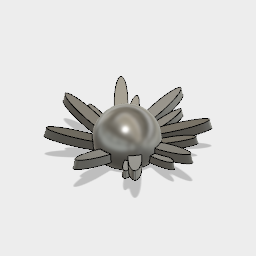
FPROJ_5 (Autodesk Fusion 360 design; units mm, degrees)
Autodesk Fusion 360 part; units mm, degrees
sketch "草图1" plane through (0, 0, 0) normal (0, 1, 0) x (1, 0, 0)
  ellipse E0 centre (0, 0) end of major axis (10, 0) minor radius 2
  line L0 (-10, 0) -> (10, 0)
  line L1 (0, -2) -> (0, 2)
extrude "拉伸1" add sketch "草图1" along normal blind 3 makes body 1
move_body "移动1" bodies 1 to x (0.965926, 0.258819, 0) y (-0.258819, 0.965926, 0) z (0, 0, 1) at (-0.3407, 2.5882, 0)
box "长方体基本要素1" add length 6 width 6 height 6 placed x (0, 1, 0) y (0, 0, 1) z (1, 0, 0) at (0, -45, -4) separate body makes body 2
move_body "移动2" bodies 2 to x (1, 0, 0) y (0, 1, 0) z (0, 0, 1) at (-21.0038, 44.4151, 0)
move_body "移动3" bodies 2 to x (1, 0, 0) y (0, 1, 0) z (0, 0, 1) at (0.0398, 0.5972, 0)
pattern_circular "C-阵列1" count 8 over 360 about axis through (-14.964, 6.0123, 2) along (0, -1, 0) of bodies 1 makes body 3 at (-1.9304, 3.2332, 13.051) makes body 4 at (-12.3658, 4.841, 13.4396) makes body 5 at (-26.015, 3.2332, 15.0336) makes body 6 at (-31.2179, 6.131, 3.4019) makes body 7 at (-27.9976, 3.2332, -9.051) makes body 8 at (-16.3658, 6.131, -14.2539) makes body 9 at (-3.9129, 3.2332, -11.0336)
copy_body "复制和粘贴实体1" bodies 6 3 7 8 4 9 1 5 makes body 10 makes body 11 makes body 12 makes body 13 makes body 14 makes body 15 makes body 16 makes body 17
move_body "移动4" bodies 10 11 12 13 14 15 16 17 to x (1, 0, 0) y (0, 1, 0) z (0, 0, 1) at (0.1831, -0.9664, -2.3123)
scale "缩放1" factor 0.8 about (-16.7809, -0.9664, -5.2762) bodies 10 15 11 12 17 16 14 13
move_body "移动5" bodies 2 to x (0.965926, 0, 0.258819) y (0, 1, 0) z (-0.258819, 0, 0.965926) at (0.0078, 0, 3.9411)
move_body "移动6" bodies 14 10 11 12 15 17 16 13 to x (1, 0, 0) y (0, 1, 0) z (0, 0, 1) at (-3, 0, 0)
move_body "移动7" bodies 6 7 5 1 3 4 9 8 to x (1, 0, 0) y (0, 1, 0) z (0, 0, 1) at (-2, 0, -1)
move_body "移动8" bodies 16 11 14 12 13 15 17 10 to x (0.984808, 0, 0.173648) y (0, 1, 0) z (-0.173648, 0, 0.984808) at (0.12, 0, 2.6288)
move_body "移动9" bodies 7 8 2 6 5 4 1 9 3 to x (1, 0, 0) y (0, 1, 0) z (0, 0, 1) at (-1, 0, -2)
move_body "移动10" bodies 4 5 6 3 7 8 9 1 to x (1, 0, 0) y (0, 1, 0) z (0, 0, 1) at (-1, 0, -1)
sphere "球体基本要素1" add diameter 20 placed x (-0.707107, 0, 0.707107) y (0.683013, 0.258819, 0.683013) z (-0.183013, 0.965926, -0.183013) at (14.9583, 8.4686, -0.5981) separate body makes body 18
move_body "MoveFace1" bodies 18 to x (1, 0, 0) y (0, 1, 0) z (0, 0, 1) at (-32.9825, -4.3347, 0) on bodies 18
combine "合并2" operation add target body 18 tool bodies 8 13 9 15 1 16 3 11 4 14 5 17 6 10 7 12
box "长方体基本要素2" add length 54 width 106 height 20 placed x (0, 0, 1) y (1, 0, 0) z (0, 1, 0) at (14, 0, 16) separate body makes body 19
move_body "移动11" bodies 19 to x (1, 0, 0) y (0, 1, 0) z (0, 0, 1) at (0, -112.011, -49.299)
move_body "移动12" bodies 19 to x (1, 0, 0) y (0, 1, 0) z (0, 0, 1) at (0, 80.8662, -92.7077)
move_body "移动13" bodies 19 to x (1, 0, 0) y (0, 1, 0) z (0, 0, 1) at (-100, 0, 90)
move_body "移动14" bodies 19 to x (1, 0, 0) y (0, 1, 0) z (0, 0, 1) at (0, 0, 10)
move_body "移动15" bodies 19 to x (1, 0, 0) y (0, 1, 0) z (0, 0, 1) at (20, 10, 0)
combine "合并3" operation cut target body 18 tool bodies 19
hidden bodies 2
